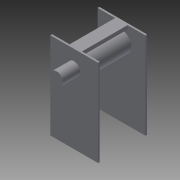
# Autodesk Inventor part: Robotics ball launcher motor frame
Saved by Autodesk Inventor 2014 (Build 180170000, 170)
## iProperties
Created: 2016-01-22
Part Number: Robotics ball launcher motor frame
Material: Generic
Document SubType Name: Modeling
Designer: shawnsargent
Density: 1 g/cm^3
Appearance: Default
Author: shawnsargent
Autodesk Inventor part; units mm, degrees
ref_plane "YZ Plane" through (0, 0, 0) normal (1, 0, 0) x (0, 1, 0)
ref_plane "XZ Plane" through (0, 0, 0) normal (0, 1, 0) x (-1, 0, 0)
ref_plane "XY Plane" through (0, 0, 0) normal (0, 0, 1) x (1, 0, 0)
sketch "Sketch1" plane through (0, 0, 0) normal (0, 0, 1) x (1, 0, 0)
  line L0 (0, 0) -> (242.2769, 0)
  line L1 (242.2769, 0) -> (242.2769, 441.325)
  line L2 (242.2769, 441.325) -> (0, 441.325)
  line L3 (0, 441.325) -> (0, 0)
  dimension "d0" = 242.2769
  dimension "d1" = 441.325
  constraints: 8 end point, 2 perpendicular, 1 horizontal, 1 parallel
  measures "d0" distance of L0.start L0.end
  measures "d1" distance of L0.end L1.end
extrude "Extrusion1" add sketch "Sketch1" along normal blind 8.7605
sketch "Sketch2" plane through (0, 0, 8.7605) normal (0, 0, 1) x (1, 0, 0)
  line L0 (242.2769, 441.325) -> (0, 441.325) projected
  line L1 (0, 441.325) -> (88.9, 441.325)
  line L2 (88.9, 441.325) -> (88.9, 422.3233)
  line L3 (88.9, 422.3233) -> (151.8437, 422.3233)
  line L4 (151.8437, 422.3233) -> (151.8437, 441.325)
  dimension "d4" = 88.9
  dimension "d5" = 19.0017
  dimension "d6" = 62.9437
  constraints: 8 end point, 2 perpendicular, 2 point on line, 1 parallel
  measures "d4" distance of L0.end L1.end
  measures "d5" distance of L1.end L2.end
  measures "d6" distance of L2.end L3.end
extrude "Extrusion2" add sketch "Sketch2" along normal blind 231.7166
sketch "Sketch3" plane through (0, 0, 240.477) normal (0, 0, 1) x (1, 0, 0)
  line L0 (88.9, 441.325) -> (88.9, 422.3233) projected
  line L1 (88.9, 422.3233) -> (151.8437, 422.3233) projected
  line L2 (151.8437, 422.3233) -> (151.8437, 441.325) projected
  line L3 (151.8437, 441.325) -> (88.9, 441.325) projected
  line L4 (88.9, 441.325) -> (0, 441.325) projected
  line L5 (151.8437, 441.325) -> (151.8437, 422.3233) projected
  line L6 (151.8437, 422.3233) -> (88.9, 422.3233) projected
  line L7 (88.9, 422.3233) -> (88.9, 441.325) projected
  line L8 (88.9, 441.325) -> (0, 441.325) projected
  line L9 (0, 441.325) -> (0, 0) projected
  line L10 (0, 0) -> (242.2769, 0) projected
  line L11 (242.2769, 0) -> (242.2769, 441.325) projected
  line L12 (242.2769, 441.325) -> (151.8437, 441.325) projected
extrude "Extrusion3" add sketch "Sketch3" along normal blind 8.7605
sketch "Sketch6" plane through (0, 0, 8.7605) normal (0, 0, 1) x (1, 0, 0)
  circle A0 centre (120.3719, 355.4324) radius 50.8
  constraints: 1 centre point
extrude "Extrusion4" add sketch "Sketch6" along normal blind 231.7166
sketch "Sketch7" plane through (0, 0, 249.2375) normal (0, 0, 1) x (1, 0, 0)
  circle A0 centre (120.3719, 355.4324) radius 50.8 projected
  circle A1 centre (120.3719, 355.4324) radius 31.75
  dimension "d15" = 63.5
  constraints: 1 centre point, 1 coincident
  measures "d15" diameter of A1
extrude "Extrusion5" add sketch "Sketch7" along normal blind 88.9 contours A1
body "Solid1"
